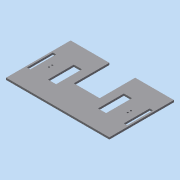
# Autodesk Inventor part: FahrwerkbasisBsp
Saved by Autodesk Inventor 2015 (Build 190159000, 159)
## iProperties
Created: 2017-11-10
Part Number: FahrwerkbasisBsp
Material: Generisch
Document SubType Name: Modeling
Designer: Christoph Soppa
Density: 1 g/cm^3
Appearance: Vorgabe
Author: Christoph Soppa
Autodesk Inventor part; units mm, degrees
ref_plane "YZ Plane" through (0, 0, 0) normal (1, 0, 0) x (0, 1, 0)
ref_plane "XZ Plane" through (0, 0, 0) normal (0, 1, 0) x (-1, 0, 0)
ref_plane "XY Plane" through (0, 0, 0) normal (0, 0, 1) x (1, 0, 0)
sketch "Skizze1" plane through (0, 0, 0) normal (0, 0, 1) x (1, 0, 0)
  line L0 (0, 0) -> (0, 200)
  line L1 (0, 200) -> (120, 200)
  line L2 (120, 200) -> (120, 90)
  line L3 (120, 90) -> (200, 90)
  line L4 (200, 90) -> (200, 200)
  line L5 (200, 200) -> (320, 200)
  line L6 (320, 200) -> (320, 0)
  line L7 (320, 0) -> (0, 0)
  line L8 (5, 60) -> (15, 60)
  line L9 (15, 60) -> (15, 140)
  line L10 (15, 140) -> (5, 140)
  line L11 (5, 140) -> (5, 60)
  line L12 (70, 140) -> (95, 140)
  line L13 (95, 140) -> (95, 60)
  line L14 (95, 60) -> (70, 60)
  line L15 (70, 60) -> (70, 140)
  line L16 (250, 140) -> (225, 140)
  line L17 (225, 140) -> (225, 60)
  line L18 (225, 60) -> (250, 60)
  line L19 (250, 60) -> (250, 140)
  line L20 (315, 140) -> (305, 140)
  line L21 (305, 140) -> (305, 60)
  line L22 (305, 60) -> (315, 60)
  line L23 (315, 60) -> (315, 140)
  dimension "d0" = 320
  dimension "d1" = 200
  dimension "d4" = 110
  dimension "d5" = 80
  dimension "d6" = 10
  dimension "d7" = 25
  dimension "d8" = 80
  dimension "d9" = 25
  dimension "d10" = 80
  dimension "d11" = 10
  dimension "d12" = 5
  dimension "d13" = 55
  dimension "d14" = 55
  dimension "d15" = 5
  dimension "d16" = 60
  dimension "d17" = 60
  dimension "d18" = 60
  dimension "d21" = 105
  dimension "d22" = 105
  constraints: 48 end point, 10 perpendicular, 8 parallel, 4 horizontal, 4 point on line, 1 vertical
  measures "d0" distance of L6.end L0.start
  measures "d1" distance of L0.start L0.end
  measures "d4" distance of L3.end L4.end
  measures "d5" distance of L8.end L9.end
  measures "d6" distance of L9.end L10.end
  measures "d7" distance of L12.start L12.end
  measures "d8" distance of L14.end L12.start
  measures "d9" distance of L16.start L16.end
  measures "d10" distance of L20.end L21.end
  measures "d11" distance of L20.start L20.end
  measures "d12" distance between parallel lines of L0 L11
  measures "d13" distance between parallel lines of L9 L15
  measures "d14" distance between parallel lines of L19 L21
  measures "d15" distance between parallel lines of L23 L6
  measures "d16" distance between parallel lines of L8 L7
  measures "d17" distance between parallel lines of L7 L22
  measures "d18" distance between parallel lines of L7 L18
  measures "d21" distance between parallel lines of L4 L21
  measures "d22" distance between parallel lines of L2 L9
extrude "Extrusion1" add sketch "Skizze1" along normal blind 6
hole "Bohrung1" at (38, 105, 6) direction (0, 0, -1) diameter 5 depth 8 tip angle 118
hole "Bohrung2" at (38, 95, 6) direction (0, 0, -1) diameter 5 depth 8 tip angle 118
hole "Bohrung5" at (282, 105, 6) direction (0, 0, -1) diameter 5 depth 8 tip angle 118
hole "Bohrung6" at (282, 95, 6) direction (0, 0, -1) diameter 5 depth 8 tip angle 118
